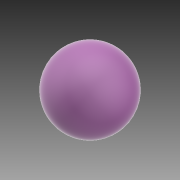
# Autodesk Inventor part: FRC 2014 Ball
Saved by Autodesk Inventor 2022 (Build 260153000, 153)
## iProperties
Created: 2021-05-01
Part Number: FRC 2014 Ball
Material: Generic
Document SubType Name: Modeling
Designer: Cal
Density: 1 g/cm^3
Appearance: Smooth - Purple
Author: Cal
Autodesk Inventor part; units mm, degrees
ref_plane "YZ Plane" through (0, 0, 0) normal (1, 0, 0) x (0, 1, 0)
ref_plane "XZ Plane" through (0, 0, 0) normal (0, 1, 0) x (-1, 0, 0)
ref_plane "XY Plane" through (0, 0, 0) normal (0, 0, 1) x (1, 0, 0)
sketch "Sketch1" plane through (0, 0, 0) normal (0, 0, 1) x (1, 0, 0)
  arc A0 (0, -304.8) -> (0, 304.8) centre (0, 0) ccw
  line L0 (0, 304.8) -> (0, -309.066)
  dimension "d0" = 609.6
  constraints: 2 end point, 2 point on circle, 2 point on line, 1 centre point, 1 coincident, 1 vertical
  measures "d0" diameter of A0
revolve "Revolution1" add sketch "Sketch1" angle 360 about axis through (0, 304.8, 0) along (0, -1, 0)
body "Solid1"
